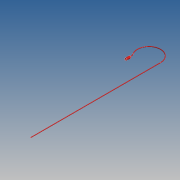
# Autodesk Inventor part: F118Laser
Saved by Autodesk Inventor 2017 (Build 210142000, 142)
## iProperties
Created: 2018-01-17
Part Number: F118Laser
Material: Générique
Document SubType Name: Modeling
Designer: serge.amoos
Density: 1 g/cm^3
Appearance: Light Red
Author: serge.amoos
Autodesk Inventor part; units mm, degrees
ref_plane "YZ Plane" through (0, 0, 0) normal (1, 0, 0) x (0, 1, 0)
ref_plane "XZ Plane" through (0, 0, 0) normal (0, 1, 0) x (-1, 0, 0)
ref_plane "XY Plane" through (0, 0, 0) normal (0, 0, 1) x (1, 0, 0)
sketch "Sketch1" plane through (0, 0, 0) normal (0, 0, 1) x (1, 0, 0)
  line L0 (-7.2, 0) -> (1.2, 0) construction
  line L1 (0, -5) -> (0, 30) construction
  line L2 (0, 0) -> (-2.5, 0)
  line L3 (-2.5, 0) -> (-2.5, 5)
  line L4 (-2.5, 5) -> (-6, 5)
  line L5 (-6, 5) -> (-6, 25)
  line L6 (-6, 25) -> (0, 25)
  line L7 (0, 25) -> (0, 0)
  dimension "d0" = 5
  dimension "d1" = 12
  dimension "d2" = 5
  dimension "d3" = 25
  constraints: 12 end point, 3 perpendicular, 2 point on line, 1 collinear, 1 vertical
  measures "d0" diameter of L3 L1
  measures "d1" diameter of L5 L1
  measures "d2" distance between parallel lines of L0 L4
  measures "d3" distance between parallel lines of L0 L6
revolve "Revolution1" add sketch "Sketch1" angle 360 about axis through (0, -10, 0) along (0, 1, 0)
sketch "Sketch2" plane through (0, 0, 0) normal (0, 0, 1) x (1, 0, 0)
  line L0 (0, -5) -> (0, 30) construction
  line L1 (6, 25) -> (-6, 25) construction
  line L2 (0, 25) -> (0, 30)
  line L3 (105.9337, -600) -> (105.9337, 80)
  arc A0 (105.9337, 80) -> (-4.9943, 46.5746) centre (45.4337, 80) ccw
  arc A1 (0, 30) -> (-4.9943, 46.5746) centre (-30, 30) ccw
  line L4 (-74.1691, 0) -> (235.0145, 0) projected
  point P0 (0, 0)
  point P1 (0, 40.0497)
  dimension "d5" = 30
  dimension "d9" = 5
  dimension "d10" = 60.5
  dimension "d11" = 80
  dimension "d12" = 600
  constraints: 5 point on circle, 4 end point, 3 tangent, 2 centre point, 2 point on line, 1 midpoint, 1 vertical
  measures "d5" radius of A1
  measures "d9" distance from line of L1 L2.end
  measures "d10" radius of A0
  measures "d11" distance from line of L4 A0.centre
  measures "d12" distance from line of L3.start L4
sketch "Sketch3" plane through (0, 25, 0) normal (0, 1, 0) x (1, 0, 0)
  circle A0 centre (0, 0) radius 1.75
  dimension "d6" = 3.5
  constraints: 1 centre point, 1 coincident
  measures "d6" diameter of A0
sweep "Sweep1" add profiles "Sketch3" path "Sketch2" path curves L2 A1 A0 L3
body "Solid1"
